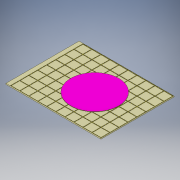
# Autodesk Inventor part: PetriFilm_Agar
Saved by Autodesk Inventor 2019 (Build 230136000, 136)
## iProperties
Created: 2019-07-12
Part Number: PetriFilm_Agar
Material: Polypropylene
Document SubType Name: Modeling
Designer: Jorian Bruslind
Density: 0.899 g/cm^3
Appearance: Smooth - Ash
Author: Jorian Bruslind
Autodesk Inventor part; units mm, degrees
ref_plane "YZ Plane" through (0, 0, 0) normal (1, 0, 0) x (0, 1, 0)
ref_plane "XZ Plane" through (0, 0, 0) normal (0, 1, 0) x (-1, 0, 0)
sketch "Sketch1" plane through (0, 0, 0) normal (0, 1, 0) x (-1, 0, 0)
  line L0 (0, 0) -> (100, 0)
  line L1 (100, 0) -> (100, -77)
  line L2 (100, -77) -> (0, -77)
  line L3 (0, -77) -> (0, 0)
  dimension "d0" = 100
  dimension "d1" = 77
  constraints: 8 end point, 2 parallel, 1 horizontal, 1 perpendicular
  measures "d0" distance of L1.end L2.end
  measures "d1" distance of L0.end L1.end
extrude "Extrusion1" add sketch "Sketch1" along normal blind 1
sketch "Sketch2" plane through (0, 1, 0) normal (0, 1, 0) x (1, 0, 0)
  line L0 (-100, 0) -> (0, 0) projected
  line L1 (0, 0) -> (-10, 0)
  line L2 (-10, 0) -> (-10, 10)
  line L3 (-10, 10) -> (0, 10)
  line L4 (0, 10) -> (0, 0)
  line L5 (-9.5, 9.5) -> (-9.5, 0.5)
  line L6 (-9.5, 0.5) -> (-0.5, 0.5)
  line L7 (-0.5, 0.5) -> (-0.5, 9.5)
  line L8 (-0.5, 9.5) -> (-9.5, 9.5)
  dimension "d4" = 10
  dimension "d5" = 10
  dimension "d6" = 0.5
  constraints: 16 end point, 4 parallel, 2 perpendicular, 1 horizontal, 3 other
  measures "d4" distance of L2.end L3.end
  measures "d5" distance of L1.end L2.end
  measures "d6" distance between parallel lines of L2 L5
extrude "Extrusion2" add sketch "Sketch2" along normal blind 0.15
pattern_linear "Rectangular Pattern1" count 10 spacing 9.5 along (-1, 0, 0) count 8 spacing 9.5 along (0, 0, -1) of "Extrusion2"
ref_plane "Work Plane1" through (0, 1.15, 0) normal (0, 1, 0) x (1, 0, 0)
sketch "Sketch4" plane through (0, 1.15, 0) normal (0, 1, 0) x (1, 0, 0)
  circle A0 centre (-45, 38.5) radius 25.2
  line L0 (0, 0) -> (0, 76.5) projected
  line L1 (0, 77) -> (-100, 77) projected
  dimension "d21" = 50.4
  dimension "d22" = 45
  dimension "d23" = 38.5
  constraints: 1 centre point
  measures "d21" diameter of A0
  measures "d22" distance from line of L0 A0.centre
  measures "d23" distance from line of L1 A0.centre
extrude "Extrusion4" add sketch "Sketch4" along normal mid plane 0.3
body "Solid1"
